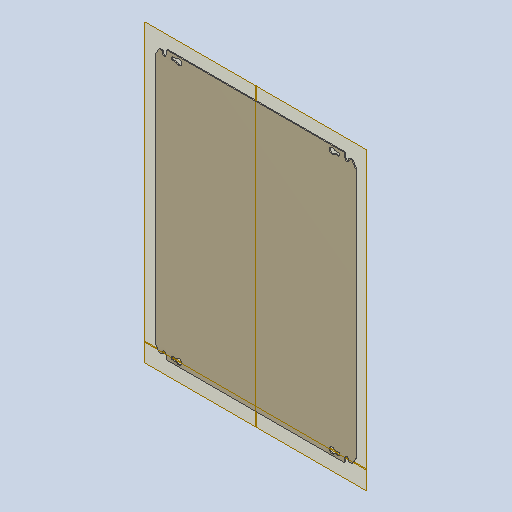
# Autodesk Inventor part: 1676X_02_00_P6_(1)
Saved by Autodesk Inventor 2025.2 (Build 292293000, 293)
## iProperties
Created: 2025-05-05
Part Number: 1676X_02_00_P6_(1)
Material: Generic
Catalog Web Link: www.cadenas.de
Description: AE 2.0 Montageplatte-AE 2.0 Montageplatte
Vendor: RITTAL
Document SubType Name: Modeling
Designer: psAdmin
Manufacturer: RITTAL
Mass: 1003.3 g
Surface Area: 8098.76 cm^2
Volume: 1003.3 cm^3
Density: 1 g/cm^3
Appearance: PSOLRGB-175-175-175
Category: PARTsolutions
Company: RITTAL
PSOL_IDENT_0: {$CADENAS_DATA/23d-libs/rittal/schaltschranksys/kompakt_schaltschr/parts_ae_2_0/montageplatte_ae_2_0
PSOL_IDENT_1: .prj},199 {VTYP=3D},{NB=1676X_02_00_P6_(1)},{LINA=1676X_02_00_P6},{NN=AE 2.0 Montageplatte},{DATE=28
PSOL_IDENT_2: .04.2025 21:11:32},{GEOMDATE=11.04.2025 07:46:14},{VERSION=},{LINEID=330},{WBVAR=DETAIL},{WBNUMERIC=
PSOL_IDENT_3: DETAIL}  {NB=1676X_02_00_P6_(1)},{LINA=1676X_02_00_P6},{KT=DUMMY},{BEST=1676X},{B=600},{H=760},{S=2.
PSOL_IDENT_4: 5},{T=MIN},{B1=550},{H1=735},{VERS=3},{DETAIL=1},{BEZ1=Neues Kompaktgehäuse},{BEZ2=Stahlblech},{BEZ3=
PSOL_IDENT_5: eintürig},{F=550},{G=735},{CNSECLASS51=27-18-01-02},{CNSECLASS70=27-18-01-01},{CNSECLASS80=27-18-01-
PSOL_IDENT_6: 01},{CNSETIM40=EC000261}
NB: 1676X_02_00_P6_(1)
NN: AE 2.0 Montageplatte
NT: AE 2.0 Montageplatte
NBSYN: $BEST._02_00_P6_($DETAIL.)
LINA: 1676X_02_00_P6
CATALOG: Rittal
BEST: 1676X
B: 600
H: 760
S: 2.5
T: 0
B1: 550
H1: 735
VERS: 3
DETAIL: hoch
BEZ1: Neues Kompaktgehäuse
BEZ2: Stahlblech
BEZ3: eintürig
F: 550
G: 735
CNSECLASS70: 27-18-01-01
CNSECLASS80: 27-18-01-01
SUPPLIER: RITTAL
ARTICLENO: 1676X_02_00_P6_(1)
BOMINFO: 1676X_02_00_P6
CREATOR: CADENAS GmbH
Title: 1676X_02_00_P6
Author: Cadenas PARTsolutions
Comments: AE 2.0 Montageplatte
Autodesk Inventor part; units mm, degrees
sketch "Sketch_11" plane through (0, 0, 0) normal (0, 0, 1) x (1, 0, 0)
  line L0 (-275, 698.5) -> (-275, 11.5)
  line L1 (-275, 11.5) -> (-274.0774, 11.5)
  arc A0 (-273.2113, 11) -> (-274.0774, 11.5) centre (-274.0774, 10.5) ccw
  line L2 (-273.2113, 11) -> (-264.2624, -4.5)
  arc A1 (-264.2624, -4.5) -> (-263.3964, -5) centre (-263.3964, -4) ccw
  line L3 (-263.3964, -5) -> (-256.5, -5)
  arc A2 (-256.5, -5) -> (-255.5, -4) centre (-256.5, -4) ccw
  line L4 (-255.5, -4) -> (-255.5, 0)
  arc A3 (-244.5, 0) -> (-255.5, 0) centre (-250, 0) ccw
  line L5 (-244.5, 0) -> (-244.5, -11)
  line L6 (-244.5, -11) -> (-243, -12.5)
  line L7 (-243, -12.5) -> (243, -12.5)
  line L8 (243, -12.5) -> (244.5, -11)
  line L9 (244.5, -11) -> (244.5, 0)
  arc A4 (255.5, 0) -> (244.5, 0) centre (250, 0) ccw
  line L10 (255.5, 0) -> (255.5, -4)
  arc A5 (255.5, -4) -> (256.5, -5) centre (256.5, -4) ccw
  line L11 (256.5, -5) -> (263.3964, -5)
  arc A6 (263.3964, -5) -> (264.2624, -4.5) centre (263.3964, -4) ccw
  line L12 (264.2624, -4.5) -> (273.2113, 11)
  arc A7 (274.0774, 11.5) -> (273.2113, 11) centre (274.0774, 10.5) ccw
  line L13 (274.0774, 11.5) -> (275, 11.5)
  line L14 (275, 11.5) -> (275, 698.5)
  line L15 (275, 698.5) -> (274.0774, 698.5)
  arc A8 (273.2113, 699) -> (274.0774, 698.5) centre (274.0774, 699.5) ccw
  line L16 (273.2113, 699) -> (264.2624, 714.5)
  arc A9 (264.2624, 714.5) -> (263.3964, 715) centre (263.3964, 714) ccw
  line L17 (263.3964, 715) -> (256.5, 715)
  arc A10 (256.5, 715) -> (255.5, 714) centre (256.5, 714) ccw
  line L18 (255.5, 714) -> (255.5, 710)
  arc A11 (244.5, 710) -> (255.5, 710) centre (250, 710) ccw
  line L19 (244.5, 710) -> (244.5, 721)
  line L20 (244.5, 721) -> (243, 722.5)
  line L21 (243, 722.5) -> (-243, 722.5)
  line L22 (-243, 722.5) -> (-244.5, 721)
  line L23 (-244.5, 721) -> (-244.5, 710)
  arc A12 (-255.5, 710) -> (-244.5, 710) centre (-250, 710) ccw
  line L24 (-255.5, 710) -> (-255.5, 714)
  arc A13 (-255.5, 714) -> (-256.5, 715) centre (-256.5, 714) ccw
  line L25 (-256.5, 715) -> (-263.3964, 715)
  arc A14 (-263.3964, 715) -> (-264.2624, 714.5) centre (-263.3964, 714) ccw
  line L26 (-264.2624, 714.5) -> (-273.2113, 699)
  arc A15 (-274.0774, 698.5) -> (-273.2113, 699) centre (-274.0774, 699.5) ccw
  line L27 (-274.0774, 698.5) -> (-275, 698.5)
  arc A16 (216.5296, 4.6222) -> (216.5296, -4.6222) centre (210, 0) ccw
  arc A17 (217.3457, -4.2) -> (216.5296, -4.6222) centre (217.3457, -5.2) ccw
  line L28 (217.3457, -4.2) -> (228, -4.2)
  arc A18 (228, -4.2) -> (229, -3.2) centre (228, -3.2) ccw
  line L29 (229, -3.2) -> (229, 3.2)
  arc A19 (229, 3.2) -> (228, 4.2) centre (228, 3.2) ccw
  line L30 (228, 4.2) -> (217.3457, 4.2)
  arc A20 (216.5296, 4.6222) -> (217.3457, 4.2) centre (217.3457, 5.2) ccw
  arc A21 (216.5296, 714.6222) -> (216.5296, 705.3778) centre (210, 710) ccw
  arc A22 (217.3457, 705.8) -> (216.5296, 705.3778) centre (217.3457, 704.8) ccw
  line L31 (217.3457, 705.8) -> (228, 705.8)
  arc A23 (228, 705.8) -> (229, 706.8) centre (228, 706.8) ccw
  line L32 (229, 706.8) -> (229, 713.2)
  arc A24 (229, 713.2) -> (228, 714.2) centre (228, 713.2) ccw
  line L33 (228, 714.2) -> (217.3457, 714.2)
  arc A25 (216.5296, 714.6222) -> (217.3457, 714.2) centre (217.3457, 715.2) ccw
  line L34 (-229, 3.2) -> (-229, -3.2)
  arc A26 (-229, -3.2) -> (-228, -4.2) centre (-228, -3.2) ccw
  line L35 (-228, -4.2) -> (-217.3457, -4.2)
  arc A27 (-216.5296, -4.6222) -> (-217.3457, -4.2) centre (-217.3457, -5.2) ccw
  arc A28 (-216.5296, -4.6222) -> (-216.5296, 4.6222) centre (-210, 0) ccw
  arc A29 (-217.3457, 4.2) -> (-216.5296, 4.6222) centre (-217.3457, 5.2) ccw
  line L36 (-217.3457, 4.2) -> (-228, 4.2)
  arc A30 (-228, 4.2) -> (-229, 3.2) centre (-228, 3.2) ccw
  arc A31 (-229, 706.8) -> (-228, 705.8) centre (-228, 706.8) ccw
  line L37 (-228, 705.8) -> (-217.3457, 705.8)
  arc A32 (-216.5296, 705.3778) -> (-217.3457, 705.8) centre (-217.3457, 704.8) ccw
  arc A33 (-216.5296, 705.3778) -> (-216.5296, 714.6222) centre (-210, 710) ccw
  arc A34 (-217.3457, 714.2) -> (-216.5296, 714.6222) centre (-217.3457, 715.2) ccw
  line L38 (-217.3457, 714.2) -> (-228, 714.2)
  arc A35 (-228, 714.2) -> (-229, 713.2) centre (-228, 713.2) ccw
  line L39 (-229, 713.2) -> (-229, 706.8)
  constraints: 80 end point, 72 point on circle, 36 centre point
extrude "Extrusion1" add sketch "Sketch_11" against normal blind 2.5
ref_plane "MP_XY" through (0, 0, 0) normal (0, 0, 1) x (1, 0, 0)
ref_plane "MP_YZ" through (0, 0, 0) normal (1, 0, 0) x (0, 1, 0)
ref_plane "MP_ZX" through (0, 0, 0) normal (0, 1, 0) x (0, 0, 1)
ref_plane "to_EB_XY" through (224.8, 0, -2.5) normal (0, 0, 1) x (1, 0, 0)
ref_plane "to_EB_YZ" through (224.8, 0, -2.5) normal (1, 0, 0) x (0, 1, 0)
ref_plane "to_EB_ZX" through (224.8, 0, -2.5) normal (0, 1, 0) x (0, 0, 1)
body "Solid1"
